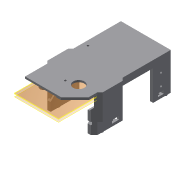
# Autodesk Inventor part: 05_Case_Bottom
Saved by Autodesk Inventor 2016 (Build 200138000, 138)
## iProperties
Created: 2016-11-09
Part Number: 05_Case_Bottom
Material: Generisch
Document SubType Name: Modeling
Designer: Bene
Density: 1 g/cm^3
Appearance: Vorgabe
Author: Bene
Autodesk Inventor part; units mm, degrees
ref_plane "Arbeitsebene1" through (0, 0, 18) normal (0, 0, 1) x (1, 0, 0)
ref_plane "Arbeitsebene2" through (0, 0, 22) normal (0, 0, 1) x (1, 0, 0)
ref_plane "Arbeitsebene4" through (0, 0, 23) normal (0, 0, 1) x (1, 0, 0)
sketch "Skizze1" plane through (0, 0, 23) normal (0, 0, 1) x (1, 0, 0)
  circle A0 centre (13.971366, 39.077453) radius 3.5 construction
  circle A1 centre (-22.528635, -44.922546) radius 3.5 construction
  circle A2 centre (-34.028634, 36.077454) radius 1.5 construction
  circle A3 centre (-4.528635, -28.922546) radius 1.5 construction
  line L0 (5.471364, -49.922547) -> (-36.528636, -49.922546) construction
  line L1 (-36.528636, -49.922546) -> (-36.528633, 73.077454) construction
  line L2 (-36.528633, 73.077454) -> (26.471367, 73.077453) construction
  line L3 (26.471367, 73.077453) -> (26.471365, -28.922547) construction
  line L4 (26.471365, -28.922547) -> (5.471364, -49.922547) construction
  line L5 (-41.528636, -54.922546) -> (7.542432, -54.922547)
  line L6 (7.542432, -54.922547) -> (31.471365, -30.993615)
  line L7 (31.471365, -30.993615) -> (31.471367, 78.077453)
  line L8 (31.471367, 78.077453) -> (-41.528633, 78.077454)
  line L9 (-41.528633, 78.077454) -> (-41.528636, -54.922546)
  circle A4 centre (-4.528635, -33) radius 1.612617
  dimension "d119" = 5
  constraints: 10 end point, 1 centre point, 4 other
  measures "d119" distance between parallel lines of L0 L5
extrude "Extrusion1" add sketch "Skizze1" along normal blind 2 contours L9 L8 L7 L6 L5 | A4
sketch "Skizze2" plane through (0, 0, 23) normal (0, 0, -1) x (-1, 0, 0)
  circle A0 centre (34.028634, 36.077454) radius 3.5
  circle A1 centre (4.528635, -28.922546) radius 3.5
  circle A2 centre (-13.971366, 39.077453) radius 4.5
  circle A3 centre (22.528635, -44.922546) radius 5.5
  circle A4 centre (-13.971366, 39.077453) radius 3.5 construction
  circle A5 centre (22.528635, -44.922546) radius 3.5 construction
  circle A6 centre (34.028634, 36.077454) radius 1.5 construction
  circle A7 centre (4.528635, -28.922546) radius 1.5 construction
  line L0 (-5.471364, -49.922547) -> (36.528636, -49.922546) construction
  line L1 (36.528636, -49.922546) -> (36.528633, 73.077454) construction
  line L2 (36.528633, 73.077454) -> (-26.471367, 73.077453) construction
  line L3 (-26.471367, 73.077453) -> (-26.471365, -28.922547) construction
  line L4 (-26.471365, -28.922547) -> (-5.471364, -49.922547) construction
  point P0 (0, 0)
  dimension "d30" = 54
  constraints: 4 centre point, 2 coincident
ref_plane "Arbeitsebene3" through (-30.289907, -72.922529, 0) normal (0, 0, 1) x (1, 0, 0)
extrude "Extrusion2" add sketch "Skizze2" along normal blind 4
sketch "Skizze3" plane through (0, 0, 25) normal (0, 0, 1) x (1, 0, 0)
  circle A0 centre (13.971366, 39.077453) radius 4.5 construction
  circle A1 centre (-22.528635, -44.922546) radius 5.5 construction
  circle A2 centre (-4.528635, -28.922546) radius 3.5 construction
  circle A3 centre (-34.028634, 36.077454) radius 3.5 construction
  line L0 (-41.528636, -54.922546) -> (7.542432, -54.922547) construction
  line L1 (-41.528633, 78.077454) -> (-41.528636, -54.922546) construction
  line L2 (31.471367, 78.077453) -> (-41.528633, 78.077454) construction
  line L3 (31.471365, -30.993615) -> (31.471367, 78.077453) construction
  line L4 (7.542432, -54.922547) -> (31.471365, -30.993615) construction
  circle A4 centre (11.471368, -23.922529) radius 4.052366 construction
  circle A5 centre (-4.528635, -28.922546) radius 1.5
  circle A6 centre (-34.028634, 36.077454) radius 1.5
  circle A7 centre (11.471368, -23.922529) radius 4.052366 construction
  circle A8 centre (11.471368, -23.922529) radius 4.052366
  point P0 (0, 0)
  dimension "d123" = 2
  dimension "d124" = 2
  constraints: 4 centre point, 2 coincident, 1 concentric
  measures "d123" radial gap between concentric circles of A2 A5
  measures "d124" radial gap between concentric circles of A3 A6
extrude "Extrusion3" cut sketch "Skizze3" against normal through all
sketch "Skizze6" plane through (0, 0, 25) normal (0, 0, 1) x (1, 0, 0)
  line L0 (-41.528633, 78.077454) -> (-41.528636, -54.922546) construction
  circle A0 centre (-34.028634, 36.077454) radius 1.5 construction
  circle A1 centre (-4.528635, -28.922546) radius 1.5 construction
  circle A2 centre (11.471368, -23.922529) radius 4.052366 construction
  line L1 (-41.528636, -54.922546) -> (7.542432, -54.922547) construction
  line L2 (7.542432, -54.922547) -> (31.471365, -30.993615) construction
  line L3 (31.471365, -30.993615) -> (31.471367, 78.077453) construction
  line L4 (31.471367, 78.077453) -> (-41.528633, 78.077454) construction
  line L5 (-41.528633, 78.077454) -> (-41.528636, -54.922546) construction
  line L6 (31.471367, 78.077453) -> (-41.528636, 78.077453) construction
  line L7 (-41.528636, 78.077453) -> (-41.528636, 95.077471) construction
  line L8 (-41.528636, 95.077471) -> (31.471367, 95.077471) construction
  line L9 (31.471367, 95.077471) -> (31.471367, 78.077453) construction
  line L10 (31.471367, 95.077471) -> (31.471365, -30.993615)
  line L11 (31.471365, -30.993615) -> (31.471367, 78.077453)
  line L12 (31.471365, -30.993615) -> (7.542432, -54.922547)
  line L13 (-41.528636, -54.922546) -> (7.542432, -54.922547)
  line L14 (7.542432, -54.922547) -> (-41.528636, -54.922546)
  line L15 (-41.528636, -54.922546) -> (-41.528636, 95.077471)
  line L16 (-41.528636, 95.077471) -> (31.471367, 95.077471)
  circle A3 centre (11.471368, -23.922529) radius 4.052366
  circle A4 centre (-34.028634, 36.077454) radius 1.5
  circle A5 centre (-4.528635, -28.922546) radius 1.5
  constraints: 18 end point, 3 perpendicular, 2 horizontal, 2 parallel, 1 vertical
extrude "Extrusion6" add sketch "Skizze6" along normal blind 4
sketch "Skizze7" plane through (0, 0, 29) normal (0, 0, 1) x (1, 0, 0)
  line L0 (-41.528636, -54.922546) -> (7.542432, -54.922547) construction
  line L1 (7.542432, -54.922547) -> (31.471365, -30.993615) construction
  line L2 (31.471365, -30.993615) -> (31.471367, 95.077471) construction
  line L3 (31.471367, 95.077471) -> (-41.528636, 95.077471) construction
  line L4 (-41.528636, 95.077471) -> (-41.528636, -54.922546) construction
  line L5 (36.471367, 100.077471) -> (36.471365, -33.064683) construction
  line L6 (36.471365, -33.064683) -> (9.6135, -59.922547) construction
  line L7 (9.6135, -59.922547) -> (-46.528636, -59.922546) construction
  line L8 (-46.528636, -59.922546) -> (-46.528636, 100.077471) construction
  line L9 (-46.528636, 100.077471) -> (36.471367, 100.077471) construction
  line L10 (31.471367, 95.077471) -> (-41.528636, 95.077471)
  line L11 (31.471367, 95.077471) -> (36.471367, 95.077471)
  line L12 (36.471367, 95.077471) -> (36.471365, -33.064683)
  line L13 (36.471365, -33.064683) -> (14.6135, -54.922547)
  line L14 (7.542432, -54.922547) -> (31.471365, -30.993615)
  line L15 (7.542432, -54.922547) -> (14.6135, -54.922547)
  line L16 (31.471365, -30.993615) -> (31.471367, 95.077471)
  line L17 (31.471365, -30.993615) -> (31.471367, 95.077471)
  dimension "d129" = 5
  constraints: 20 end point, 3 perpendicular, 2 point on line, 1 vertical, 4 other
  measures "d129" distance between parallel lines of L2 L5
extrude "Extrusion7" add sketch "Skizze7" against normal up to surface (4 mm away)
sketch "Skizze8" plane through (0, 0, 25) normal (0, 0, -1) x (-1, 0, 0)
  line L0 (-31.471367, 78.077453) -> (41.528633, 78.077454) construction
  line L1 (41.528636, 95.077471) -> (41.528633, 78.077454) construction
  line L2 (-31.471365, -30.993615) -> (-31.471367, 78.077453) construction
  line L3 (-31.471367, 78.077453) -> (41.528633, 78.077454) construction
  line L4 (-36.471368, 95.077471) -> (-28.471368, 95.077471)
  line L5 (-28.471368, 95.077471) -> (-28.471368, 78.077453)
  line L6 (-28.471368, 78.077453) -> (-36.471368, 78.077453)
  line L7 (-36.471368, 78.077453) -> (-36.471368, 95.077471)
  line L8 (-31.471368, 95.077471) -> (41.528636, 95.077471) construction
  line L9 (24.528632, 95.077471) -> (16.528632, 95.077471)
  line L10 (16.528632, 95.077471) -> (16.528632, 78.077454)
  line L11 (16.528632, 78.077454) -> (24.528632, 78.077454)
  line L12 (24.528632, 78.077454) -> (24.528632, 95.077471)
  line L13 (-31.471367, 95.077471) -> (41.528636, 95.077471)
  line L14 (-36.471367, 95.077471) -> (-36.471365, -33.064683)
  line L15 (-36.471365, -33.064683) -> (-14.6135, -54.922547)
  line L16 (-14.6135, -54.922547) -> (-7.542432, -54.922547)
  line L17 (-31.471365, -30.993615) -> (-7.542432, -54.922547)
  line L18 (-31.471367, 95.077471) -> (-36.471367, 95.077471)
  line L19 (-36.471368, 78.077453) -> (-28.471368, 78.077453)
  line L20 (-28.471368, 78.077453) -> (-28.471368, 74.077453)
  line L21 (-28.471368, 74.077453) -> (-36.471368, 74.077453)
  line L22 (-36.471368, 74.077453) -> (-36.471368, 78.077453)
  line L23 (16.528632, 78.077454) -> (24.528632, 78.077454)
  line L24 (24.528632, 78.077454) -> (24.528632, 74.077454)
  line L25 (24.528632, 74.077454) -> (16.528632, 74.077454)
  line L26 (16.528632, 74.077454) -> (16.528632, 78.077454)
  line L27 (-36.471368, 78.077453) -> (-31.471366, 78.077453)
  line L28 (-31.471366, 78.077453) -> (-31.471366, 67.492381)
  line L29 (-31.471366, 67.492381) -> (-36.471368, 67.492381)
  line L30 (-36.471368, 67.492381) -> (-36.471368, 78.077453)
  dimension "d126" = 8
  dimension "d127" = 8
  dimension "d128" = 45
  dimension "d225" = 4
  dimension "d226" = 4
  constraints: 40 end point, 10 parallel, 5 horizontal, 5 perpendicular, 4 point on line
  measures "d126" distance of L5.end L6.end
  measures "d127" distance of L11.end L10.end
  measures "d128" distance between parallel lines of L5 L10
  measures "d225" distance of L19.end L20.end
  measures "d226" distance of L23.end L24.end
ref_plane "Arbeitsebene5" through (-15.028632, 71.077471, -46) normal (0, 0, -1) x (0, 1, 0)
extrude "Extrusion8" add sketch "Skizze8" along normal blind 54 contours L4 L5 L6 L7 | L6 L28 L21 L14 | L21 L28 L29 L14 | L12 L11 L10 L9 | L24 L25 L26 L11
sketch "Skizze12" plane through (0, 0, 29) normal (0, 0, 1) x (1, 0, 0)
  line L0 (36.471368, 20.077471) -> (32.077024, 20.077471)
  line L1 (26.471368, 16.55369) -> (26.471368, -14.922529)
  line L2 (26.471368, -14.922529) -> (36.471368, -14.922529)
  line L3 (36.471368, -14.922529) -> (36.471368, 20.077471)
  line L4 (-41.528632, -14.922529) -> (-31.528632, -14.922529)
  line L5 (-31.528632, -14.922529) -> (-31.528632, 20.077471)
  line L6 (-31.528632, 20.077471) -> (-41.528632, 20.077471)
  line L7 (-41.528632, 20.077471) -> (-41.528632, -14.922529)
  line L8 (26.471368, 16.55369) -> (33.471368, 16.55369)
  line L9 (33.471368, 16.55369) -> (33.471368, 12.55369)
  line L10 (33.471368, 12.55369) -> (26.471368, 12.55369)
  line L11 (26.471368, 12.55369) -> (26.471368, 16.55369)
  line L12 (-31.528632, 16.55369) -> (-39.048055, 16.55369)
  line L13 (-39.048055, 16.55369) -> (-39.048055, 12.55369)
  line L14 (-39.048055, 12.55369) -> (-31.528632, 12.55369)
  line L15 (-31.528632, 12.55369) -> (-31.528632, 16.55369)
  line L16 (-30.528632, 13.077471) -> (19.471368, 13.077471) construction
  line L17 (-30.528632, 16.077471) -> (-30.528632, 13.077471) construction
  line L18 (19.471368, 16.077471) -> (-30.528632, 16.077471) construction
  line L19 (19.471368, 16.077471) -> (19.471368, 13.077471) construction
  line L20 (33.471368, 16.55369) -> (32.077024, 20.077471)
  line L21 (-41.528632, -14.922529) -> (-31.528632, -14.922529)
  line L22 (-31.528632, -14.922529) -> (-31.528632, -24.922529)
  line L23 (-31.528632, -24.922529) -> (-41.528632, -24.922529)
  line L24 (-41.528632, -24.922529) -> (-41.528632, -14.922529)
  line L25 (26.471368, -14.922529) -> (36.471368, -14.922529)
  line L26 (36.471368, -14.922529) -> (36.471368, -24.922529)
  line L27 (36.471368, -24.922529) -> (26.471368, -24.922529)
  line L28 (26.471368, -24.922529) -> (26.471368, -14.922529)
  dimension "d43" = 10
  dimension "d45" = 10
  dimension "d46" = 7
  dimension "d50" = 35
  dimension "d51" = 0
  dimension "d130" = 35
  dimension "d131" = 4
  dimension "d132" = 4
  dimension "d133" = 4
  dimension "d200" = 10
  dimension "d201" = 10
  dimension "d202" = 10
  dimension "d203" = 10
  constraints: 50 end point, 12 parallel, 6 horizontal, 6 perpendicular, 2 point on line
  measures "d43" distance of L2.end L1.end
  measures "d45" distance of L6.end L5.end
  measures "d46" distance of L9.end L10.end
  measures "d50" distance between parallel lines of L4 L6
  measures "d51" distance between parallel lines of L2 L4
  measures "d130" distance between parallel lines of L2 L0
  measures "d131" distance between parallel lines of L6 L18
  measures "d132" distance between parallel lines of L10 L8
  measures "d133" distance between parallel lines of L14 L12
  measures "d200" distance of L22.end L23.end
  measures "d201" distance of L21.end L22.end
  measures "d202" distance of L26.end L27.end
  measures "d203" distance of L25.end L26.end
extrude "Extrusion11" add sketch "Skizze12" against normal up to surface (58 mm away) contours L3 L2 L1 L10 L9 L20 L0 | L26 L27 L28 L2 | L7 L6 L5 L12 L13 L14 L4 | L4 L22 L23 L24
ref_plane "Arbeitsebene6" through (-39.528632, -47.038131, -39.701388) normal (-1, 0, 0) x (0, 0, 1)
sketch "Skizze27" plane through (0, 0, -29) normal (0, 0, -1) x (-1, 0, 0)
  line L0 (24.528632, 95.077471) -> (16.528632, 95.077471)
  line L1 (16.528632, 95.077471) -> (16.528632, 74.077454)
  line L2 (24.528632, 74.077454) -> (24.528632, 95.077471)
  line L3 (-28.471368, 95.077471) -> (-36.471368, 95.077471)
  line L4 (-36.471368, 95.077471) -> (-36.471368, 67.492381)
  line L5 (-28.471368, 78.077453) -> (-28.471368, 95.077471)
  circle A0 centre (36.528632, -9.922529) radius 4
  circle A1 centre (-31.471368, -9.922529) radius 4
  circle A2 centre (-227.299575, 545.805571) radius 1.75
  circle A3 centre (-32.471368, 79.077471) radius 1.75
  circle A4 centre (20.528632, 79.077471) radius 1.75
  line L6 (38.528632, -8.400359) -> (-33.471368, -8.400359)
  circle A5 centre (-31.471365, 7.55369) radius 1.75
  line L7 (-33.471368, 12.55369) -> (-26.471368, 12.55369)
  circle A6 centre (36.528632, 9.30369) radius 1.75
  circle A7 centre (-32.471368, 79.077471) radius 2.25
  circle A8 centre (20.528632, 79.077471) radius 2.25
  line L8 (16.528632, 74.077454) -> (24.528632, 74.077454)
  line L9 (-31.471366, 78.077453) -> (-28.471368, 78.077453)
  line L10 (-36.471368, 67.492381) -> (-31.471366, 67.492381)
  line L11 (-31.471366, 67.492381) -> (-31.471366, 78.077453)
  point P0 (0, 0)
  point P1 (31.528632, -8.400359)
  dimension "d156" = 3.5
  dimension "d157" = 3.5
  dimension "d159" = 3.5
  dimension "d161" = 3.5
  dimension "d162" = 5
  dimension "d163" = 3.5
  dimension "d192" = 4
  dimension "d193" = 4
  dimension "d223" = 0
  dimension "d224" = 0
  constraints: 5 centre point
  measures "d156" diameter of A2
  measures "d157" diameter of A3
  measures "d159" diameter of A4
  measures "d161" diameter of A5
  measures "d162" distance from line of A5.centre L7
  measures "d163" diameter of A6
  measures "d192" distance from line of A4.centre L1
  measures "d193" distance from line of A3.centre L4
  measures "d223" distance of A7.centre A3.centre
  measures "d224" distance of A8.centre A4.centre
extrude "Extrusion23" cut sketch "Skizze27" against normal blind 15 contours L9 L11 A3 | A3 L11 L9 | A4 | A5 | A6
sketch "Skizze29" plane through (0, 0, 25) normal (0, 0, -1) x (-1, 0, 0)
  line L0 (-36.471368, 20.077471) -> (-32.077024, 20.077471)
  line L1 (-31.471365, -30.993615) -> (-31.471365, -24.922529)
  line L2 (-36.471368, 67.492381) -> (-36.471368, 20.077471)
  line L3 (-36.471365, -33.064683) -> (-14.6135, -54.922547)
  line L4 (-14.6135, -54.922547) -> (-7.542432, -54.922547)
  line L5 (-31.471365, -30.993615) -> (-7.542432, -54.922547)
  line L6 (-33.471368, 12.55369) -> (-31.471366, 12.55369)
  line L7 (-32.077024, 20.077471) -> (-33.471368, 16.55369)
  line L8 (-33.471368, 16.55369) -> (-33.471368, 12.55369)
  line L9 (-31.471365, -24.922529) -> (-36.471368, -24.922529)
  line L10 (-36.471368, -24.922529) -> (-36.471365, -33.064683)
  line L11 (24.528632, 78.077454) -> (41.528633, 78.077454)
  line L12 (16.528632, 78.077454) -> (16.528632, 95.077471)
  line L13 (24.528632, 95.077471) -> (41.528636, 95.077471)
  line L14 (24.528632, 95.077471) -> (24.528632, 78.077454)
  line L15 (41.528636, 95.077471) -> (41.528633, 78.077454)
  line L16 (-28.471368, 95.077471) -> (-28.471368, 78.077453)
  line L17 (-28.471368, 95.077471) -> (16.528632, 95.077471)
  line L18 (-31.471366, 12.55369) -> (-31.471366, 67.492381)
  line L19 (-31.471366, 67.492381) -> (-36.471368, 67.492381)
  line L20 (-28.471368, 78.077453) -> (16.528632, 78.077454)
  point P0 (0, 0)
extrude "Extrusion25" add sketch "Skizze29" along normal blind 7 contours L2 L19 L18 L6 L8 L7 L0
chamfer "Fase6" distance 5 angle 45 4 edges at (-24.5286, 86.5775, 25) (36.4714, -24.9225, -2) (-41.5286, -24.9225, 24) (-41.5286, -24.9225, -3)
sketch "Skizze34" plane through (26.471368, -24.922529, -29) normal (0, -1, 0) x (1, 0, 0)
  line L0 (0, 52) -> (0, 0) construction
  line L1 (0, 0) -> (5, 0) construction
  line L2 (0, 52) -> (4.999997, 52) construction
  line L3 (-58, 52) -> (-58, 0) construction
  line L4 (-63, 52) -> (-58, 52) construction
  line L5 (-63, 0) -> (-58, 0) construction
  line L6 (7.499997, 52) -> (-63, 52)
  line L7 (-63, 52) -> (-63, 32)
  line L8 (-63, 32) -> (7.499997, 32)
  line L9 (7.499997, 32) -> (7.499997, 52)
  line L10 (4.999997, 52) -> (5, 0)
  line L11 (-63, 0) -> (-63, 52)
  point P0 (-26.471368, 29)
  dimension "d206" = 20
  constraints: 8 end point, 2 parallel, 1 horizontal, 1 perpendicular, 1 point on line
  measures "d206" distance between parallel lines of L6 L8
extrude "Extrusion30" cut sketch "Skizze34" against normal up to surface (45 mm away)
chamfer "Fase7" distance 5 angle 45 2 edges at (33.9714, -1.1725, 3) (-36.5286, -6.1844, 3)
chamfer "Fase8" distance 5 angle 60 1 edges at (26.4714, 12.5537, -13) measured on face at (29.638, 12.5537, -18.3333)
sketch "Skizze38" plane through (-24.528632, 78.077453, -29) normal (-1, 0, 0) x (0, 0, 1)
  circle A0 centre (40, 5.999999) radius 1.5
  circle A1 centre (58.5, 5.999999) radius 1.5
  line L0 (49, 17.000018) -> (49, -3.999999)
  line L1 (49, 17.000018) -> (0, 17.000018)
  line L2 (0, -3.999999) -> (0, 17.000018)
  circle A2 centre (40, 5.999999) radius 1.5
  circle A3 centre (58.5, 5.999999) radius 1.5
  circle A4 centre (16.48442, 2.000018) radius 1.5
  circle A5 centre (34.960995, 2.000018) radius 1.5
  line L3 (49, -3.999999) -> (0, -3.999999)
  line L4 (16.48442, 2.000018) -> (25.426796, 2.000018) construction
  line L5 (16.48442, 3.500018) -> (25.426796, 3.500018)
  line L6 (25.426796, 0.500018) -> (16.48442, 0.500018)
  arc A6 (16.48442, 3.500018) -> (16.48442, 0.500018) centre (16.48442, 2.000018) ccw
  arc A7 (25.426796, 0.500018) -> (25.426796, 3.500018) centre (25.426796, 2.000018) ccw
  line L7 (16.48442, 2.000018) -> (10, 2.000018) construction
  line L8 (16.48442, 0.500018) -> (10, 0.500018)
  line L9 (10, 3.500018) -> (16.48442, 3.500018)
  arc A8 (16.48442, 0.500018) -> (16.48442, 3.500018) centre (16.48442, 2.000018) ccw
  arc A9 (10, 3.500018) -> (10, 0.500018) centre (10, 2.000018) ccw
  line L10 (34.960995, 2.000018) -> (41, 2) construction
  line L11 (34.960991, 0.500018) -> (40.999996, 0.5)
  line L12 (41.000004, 3.5) -> (34.961, 3.500018)
  arc A10 (34.961, 3.500018) -> (34.960991, 0.500018) centre (34.960995, 2.000018) ccw
  arc A11 (40.999996, 0.5) -> (41.000004, 3.5) centre (41, 2) ccw
  point P0 (29, -78.077453)
  point P1 (20.955608, 2.000018)
  point P2 (13.24221, 2.000018)
  point P3 (37.980498, 2.000009)
  dimension "d219" = 3
  dimension "d220" = 3
  constraints: 24 end point, 12 point on circle, 12 tangent, 10 centre point, 3 concentric, 3 midpoint, 3 parallel, 2 coincident, 1 horizontal, 1 point on line
  measures "d219" diameter of A4
  measures "d220" diameter of A5
extrude "Extrusion33" cut sketch "Skizze38" against normal through all contours A4 | A5
sketch "Skizze39" plane through (-31.528632, -24.922529, -29) normal (1, 0, 0) x (0, 0, -1)
  line L0 (-12.850192, -1.149825) -> (-14.264405, -2.564039)
  line L1 (-44.902221, 27.36667) -> (-42.780901, 29.487991)
  line L2 (-35.87868, 22.585769) -> (-12.143085, -1.149825)
  line L3 (-12.143085, -1.149825) -> (-14.264405, -3.271146)
  line L4 (-14.264405, -3.271146) -> (-38, 20.464449)
  line L5 (-38, 20.464449) -> (-35.87868, 22.585769)
  line L6 (-31.710942, 14.17539) -> (-29.589621, 16.296711)
  line L7 (-31.710942, 14.17539) -> (-28.710942, 14.17539) construction
  point P0 (-29, 24.922529)
  point P1 (-37.646447, 20.818002)
  point P2 (-36.232233, 22.232216)
  point P3 (-38, 20.464449)
  dimension "d232" = 45
  constraints: 16 end point, 4 point on line, 2 coincident, 2 parallel, 2 perpendicular, 1 equal length, 1 horizontal, 2 other
  measures "d232" angle of L7 L6
extrude "Extrusion34" cut sketch "Skizze39" along normal blind 64 and the other way blind 5
sketch "Skizze40" plane through (0, 0, 23) normal (0, 0, -1) x (-1, 0, 0)
  circle A0 centre (-13.971366, 39.077453) radius 4.5
  circle A1 centre (34.028634, 36.077454) radius 3.5
  circle A2 centre (4.528635, -28.922546) radius 3.5
  circle A3 centre (22.528635, -44.922546) radius 5.5
  line L0 (36.528632, 12.55369) -> (39.048055, 12.55369)
  line L1 (39.048055, 12.55369) -> (39.048055, 16.55369)
  line L2 (39.048055, 16.55369) -> (36.528632, 16.55369)
  line L3 (36.528632, 16.55369) -> (36.528632, 20.077471)
  line L4 (36.528632, 20.077471) -> (41.528632, 20.077471)
  line L5 (41.528633, 78.077454) -> (41.528632, 20.077471)
  line L6 (27.528632, 78.077454) -> (41.528633, 78.077454)
  line L7 (27.528632, 78.077454) -> (27.528632, 74.077454)
  line L8 (27.528632, 74.077454) -> (16.528632, 74.077454)
  line L9 (16.528632, 74.077454) -> (16.528632, 78.077454)
  line L10 (-28.471368, 78.077453) -> (16.528632, 78.077454)
  line L11 (-31.471367, 78.077453) -> (-28.471368, 78.077453)
  line L12 (-33.971365, 20.077471) -> (-31.471366, 20.077471)
  line L13 (-33.971365, -22.422532) -> (-33.971365, 20.077471)
  line L14 (-31.471365, -24.922529) -> (-33.971365, -22.422532)
  line L15 (-31.471365, -30.993615) -> (-31.471365, -24.922529)
  line L16 (-7.542432, -54.922547) -> (-31.471365, -30.993615)
  line L17 (41.528636, -54.922546) -> (-7.542432, -54.922547)
  line L18 (41.528635, -19.922529) -> (41.528636, -54.922546)
  line L19 (41.528635, -19.922529) -> (36.528632, -24.922529)
  line L20 (36.528632, -24.922529) -> (36.528632, 12.55369)
  line L21 (-31.471366, 67.492381) -> (-31.471367, 78.077453)
  line L22 (-31.471366, 20.077471) -> (-31.471366, 67.492381)
  point P0 (0, 0)
  dimension "d30" = 54
extrude "Extrusion37" cut sketch "Skizze40" against normal blind 3
sketch "Skizze41" plane through (0, 0, 26) normal (0, 0, -1) x (-1, 0, 0)
  circle A0 centre (-11.471368, -23.922529) radius 4.052366
  circle A1 centre (-11.471368, -23.922529) radius 8.772397
  point P0 (0, 0)
  constraints: 1 centre point, 1 coincident
extrude "Extrusion38" cut sketch "Skizze41" against normal blind 3
sketch "Skizze42" plane through (0, 0, 29) normal (0, 0, 1) x (1, 0, 0)
  line L0 (-41.528635, -19.922529) -> (-41.528635, -19.922529)
  line L1 (-41.528632, 20.077471) -> (-41.528635, -19.922529)
  line L2 (-41.528635, -19.922529) -> (-45.528635, -15.922528)
  line L3 (-45.528635, -15.922528) -> (-45.528632, 16.077472)
  line L4 (-45.528632, 16.077472) -> (-41.528632, 20.077471)
  line L5 (-41.528635, -19.922529) -> (-41.528632, 20.077471)
  line L6 (36.471368, -19.922529) -> (36.471368, 20.077471)
  line L7 (36.471368, -19.922529) -> (40.743868, -15.650029)
  line L8 (40.743868, -15.650029) -> (40.743868, 15.804971)
  line L9 (40.743868, 15.804971) -> (36.471368, 20.077471)
  line L10 (36.471368, 20.077471) -> (36.471368, -19.922529)
  point P0 (0, 0)
  dimension "d241" = 135
  dimension "d242" = 4
  dimension "d243" = 45
  dimension "d244" = 45
  constraints: 16 end point, 3 parallel, 1 perpendicular, 1 vertical
  measures "d241" angle of L1 L2
  measures "d242" distance between parallel lines of L1 L3
  measures "d243" angle of L7 L6
  measures "d244" angle of L6 L9
extrude "Extrusion39" add sketch "Skizze42" against normal blind 40
sketch "Skizze43" plane through (-41.528632, -19.922529, -29) normal (-1, 0, 0) x (0, 0, 1)
  line L0 (15, 27.476219) -> (15, 30.976219)
  line L1 (0, 27.476219) -> (0, 30.976219)
  line L2 (15, 25.726219) -> (15, 29.226219)
  line L3 (0, 25.726219) -> (0, 29.226219)
  line L4 (15, 100.215632) -> (15, 100.215632)
  line L5 (15, 99.784367) -> (15, 97.999982)
  line L6 (0, 97.999982) -> (15, 97.999982)
  line L7 (0, 97.56386) -> (0, 97.999982)
  line L8 (15, 97.56386) -> (0, 97.56386)
  line L9 (15, 97.56386) -> (15, 99.784367)
  line L10 (0, 97.25) -> (0, 100.75)
  line L11 (15, 100.215632) -> (15, 100.215632)
  line L12 (15, 99.784367) -> (15, 99.784367)
  line L13 (4, 23) -> (9, 23)
  line L14 (9, 23) -> (9, 34)
  line L15 (9, 34) -> (4, 34)
  line L16 (4, 34) -> (4, 23)
  line L17 (4, 95) -> (9, 95)
  line L18 (9, 95) -> (9, 104)
  line L19 (9, 104) -> (4, 104)
  line L20 (4, 104) -> (4, 95)
  point P0 (29, 19.922529)
  constraints: 16 end point, 4 parallel, 4 vertical alignment, 2 horizontal, 2 perpendicular, 2 point on line
extrude "Extrusion40" cut sketch "Skizze43" against normal through all contours L20 L19 L18 L6 | L6 L18 L8 L20 | L8 L18 L17 L20 | L16 L15 L14 L13
sketch "Skizze44" plane through (0, 0, -29) normal (0, 0, -1) x (-1, 0, 0)
  circle A0 centre (-32.471368, 90.077471) radius 3.5
  circle A1 centre (20.528632, 90.077471) radius 3.5
  circle A2 centre (-31.471368, -9.922529) radius 4.25
  circle A3 centre (36.528632, -9.922529) radius 4.25
  circle A4 centre (20.528632, 90.077471) radius 3
  circle A5 centre (-32.471368, 90.077471) radius 3
  circle A6 centre (-31.471368, -9.922529) radius 3.75
  circle A7 centre (36.528632, -9.922529) radius 3.75
  point P0 (0, 0)
  dimension "d249" = 0.5
  dimension "d250" = 0.5
  dimension "d251" = 0.5
  dimension "d252" = 0.5
  constraints: 8 centre point, 8 other
  measures "d249" radial gap between concentric circles of A1 A4
  measures "d250" radial gap between concentric circles of A0 A5
  measures "d251" radial gap between concentric circles of A3 A7
  measures "d252" radial gap between concentric circles of A2 A6
extrude "Extrusion41" add sketch "Skizze44" along normal blind 2 contours A4 | A5 | A6 | A7
